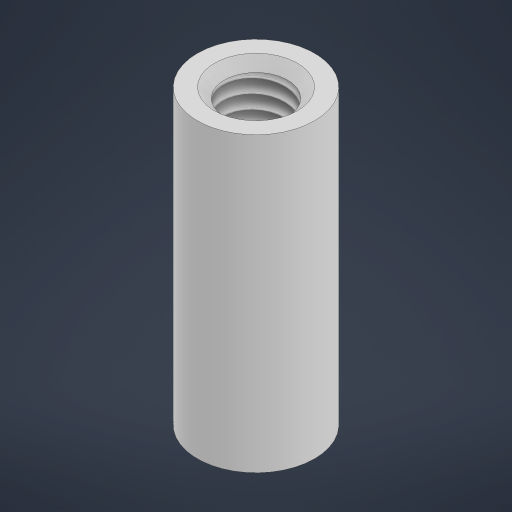
# Autodesk Inventor part: Standoff_GB
Saved by Autodesk Inventor 2024.2 (Build 282272000, 272)
## iProperties
Created: 2026-01-04
Part Number: Standoff_GB
Material: Generic
Document SubType Name: Modeling
Designer: 4aida
Density: 1 g/cm^3
Appearance: Default
Author: 4aida
Autodesk Inventor part; units mm, degrees
ref_plane "YZ Plane" through (0, 0, 0) normal (1, 0, 0) x (0, 1, 0)
ref_plane "XZ Plane" through (0, 0, 0) normal (0, 1, 0) x (-1, 0, 0)
ref_plane "XY Plane" through (0, 0, 0) normal (0, 0, 1) x (1, 0, 0)
sketch "Sketch1" plane through (0, 0, 0) normal (0, 1, 0) x (-1, 0, 0)
  circle A0 centre (0, 0) radius 3
  dimension "d0" = 6
  constraints: 1 centre point, 1 coincident
  measures "d0" diameter of A0
extrude "Extrusion1" add sketch "Sketch1" along normal mid plane 15
sketch "Sketch2" plane through (0, 7.5, 0) normal (0, 1, 0) x (1, 0, 0)
  point P0 (0, 0)
  point P1 (0, 0)
  constraints: 1 coincident
hole "Hole1" at (0, 7.5, 0) direction (0, -1, 0) diameter 3.242 depth 15 thread size "M4x0.7" class "6H" standard "ANSI Metric M Profile"
chamfer "Chamfer1" distance 0.5 angle 45 2 edges at (0, 7.5, -1.621) (0, -7.5, -1.621)
body "Solid1"
